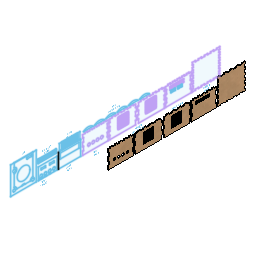
cardboard_box_v3 (Autodesk Fusion 360 design; units mm, degrees)
Autodesk Fusion 360 part; units mm, degrees
(part 1 of 3)
sketch "bottom sketch" plane through (0, 0, 0) normal (0, 0, 1) x (1, 0, 0)
  line L0 (0, 0) -> (150, 0)
  line L1 (150, 0) -> (150, 161)
  line L2 (150, 161) -> (0, 161)
  line L3 (0, 161) -> (0, 0)
  dimension "d9" = 150
  dimension "d10" = 161
  constraint horizontal L0
  constraint vertical L1
  constraint horizontal L2
  constraint vertical L3
  constraint coincident L0.start L3.end
  measures "d9" distance of L0.start L0.end
  measures "d10" distance of L0.start L2.end
extrude "Extrude1" add sketch "bottom sketch" along normal blind 5 makes body 1
sketch "bottom panel front fingers sketch" plane through (0, 0, 0) normal (0, -1, 0) x (1, 0, 0)
  line L0 (0, 0) -> (150, 0)
  line L1 (150, 0) -> (150, 5)
  line L2 (150, 5) -> (0, 5)
  line L3 (0, 5) -> (0, 0)
  line L4 (13.6364, 0) -> (27.2727, 0)
  line L5 (27.2727, 0) -> (27.2727, 5)
  line L6 (27.2727, 5) -> (13.6364, 5)
  line L7 (13.6364, 5) -> (13.6364, 0)
  dimension "d19" = 13.6364
  dimension "d20" = 13.6364
  constraint horizontal L4
  constraint vertical L5
  constraint horizontal L6
  constraint vertical L7
  constraint coincident L2 L5.end
  constraint coincident L0 L4.start
  measures "d19" distance of L5.end L6.end
  measures "d20" distance of L3 L7
extrude "Extrude2" cut sketch "bottom panel front fingers sketch" against normal blind 5 contours L0 L2 L4 L5 L6 L7 bodies 1
pattern_linear "R-Pattern1" count 5 spacing 27.2727 along (1, 0, 0) of "Extrude2"
sketch "front panel sketch" plane through (0, 0, 0) normal (0, 1, 0) x (1, 0, 0)
  line L0 (0, 0) -> (150, 0)
  line L1 (150, 0) -> (150, -110)
  line L2 (150, -110) -> (0, -110)
  line L3 (0, -110) -> (0, 0)
  dimension "d27" = 110
  constraint perpendicular L0 L1
  constraint parallel L0 L2
  constraint parallel L1 L3
  constraint horizontal L0
  constraint coincident L0.start L3.end
  measures "d27" distance of L0.start L2.end
extrude "Extrude3" add sketch "front panel sketch" along normal blind 5 separate body makes body 2
combine "Combine1" operation cut target body 2 tool bodies 1 keep tools
sketch "front panel left finger sketch" plane through (0, 0, 0) normal (-1, 0, 0) x (0, -1, 0)
  line L0 (-5, 5) -> (0, 5)
  line L1 (0, 5) -> (0, 110)
  line L2 (0, 110) -> (-5, 110)
  line L3 (-5, 110) -> (-5, 5)
  line L4 (0, 22) -> (-5, 22)
  line L5 (-5, 22) -> (-5, 44)
  line L6 (-5, 44) -> (0, 44)
  line L7 (0, 44) -> (0, 22)
  dimension "d30" = 22
  dimension "d31" = 22
  constraint horizontal L4
  constraint vertical L5
  constraint horizontal L6
  constraint vertical L7
  constraint coincident L3 L5.end
  constraint coincident L1 L4.start
  measures "d30" distance of L4.start L6.end
  measures "d31" distance of L4.start origin
extrude "Extrude4" cut sketch "front panel left finger sketch" against normal blind 5 contours L1 L3 L4 L5 L6 L7 bodies 2
pattern_linear "R-Pattern2" count 1 spacing 0 along (1, 0, 0) count 2 spacing 44 along (0, 0, 1) of "Extrude4"
extrude "Extrude5" add 1 faces at (78.9394, 5, 67.6667) along direction (0, -1, 0) blind 5 from surface at -156 separate body on bodies 2 makes body 3
combine "Combine2" operation cut target body 1 tool bodies 3 keep tools
sketch "left panel sketch" plane through (0, 0, 0) normal (1, 0, 0) x (0, 1, 0)
  line L0 (161, 0) -> (0, 0)
  line L1 (0, 0) -> (0, 110)
  line L2 (0, 110) -> (161, 110)
  line L3 (161, 110) -> (161, 0)
  line L4 (107.3333, 82.5) -> (101.3333, 82.5)
  line L5 (101.3333, 82.5) -> (101.3333, 76.5)
  line L6 (101.3333, 76.5) -> (107.3333, 76.5)
  line L7 (107.3333, 76.5) -> (107.3333, 82.5)
  dimension "d54" = 161
  dimension "d55" = 6
  dimension "d56" = 6
  dimension "d57" = 53.6667
  dimension "d66" = 27.5
  constraint perpendicular L0 L1
  constraint parallel L0 L2
  constraint parallel L1 L3
  constraint coincident L0.end L1.start
  constraint horizontal L0
  constraint horizontal L4
  constraint vertical L5
  constraint horizontal L6
  constraint vertical L7
  measures "d54" distance of L1.end L2.end
  measures "d55" distance of L4.start L4.end
  measures "d56" distance of L4.start L6.end
  measures "d57" distance of L3 L7
  measures "d66" distance of L2 L4
extrude "Extrude6" add sketch "left panel sketch" along normal blind 5 separate body contours L0 L1 L2 L3 | L4 L5 L6 L7 makes body 4
sketch "bottom panel left finger sketch" plane through (0, 0, 0) normal (-1, 0, 0) x (0, -1, 0)
  line L0 (-161, 0) -> (0, 0)
  line L1 (0, 0) -> (0, 5)
  line L2 (0, 5) -> (-161, 5)
  line L3 (-161, 5) -> (-161, 0)
  line L4 (-35.7778, 0) -> (-17.8889, 0)
  line L5 (-17.8889, 0) -> (-17.8889, 5)
  line L6 (-17.8889, 5) -> (-35.7778, 5)
  line L7 (-35.7778, 5) -> (-35.7778, 0)
  dimension "d43" = 17.8889
  dimension "d44" = 17.8889
  constraint horizontal L4
  constraint vertical L5
  constraint horizontal L6
  constraint vertical L7
  constraint coincident L2 L5.end
  constraint coincident L0 L4.start
  measures "d43" distance of L4.start L4.end
  measures "d44" distance of L1 L5
extrude "Extrude7" cut sketch "bottom panel left finger sketch" against normal blind 5 contours L0 L2 L4 L5 L6 L7 bodies 1
pattern_linear "R-Pattern3" count 4 spacing 35.7778 along (0, 1, 0) of "Extrude7"
combine "Combine3" operation cut target body 4 tool bodies 2 1 3 keep tools
extrude "Extrude9" cut sketch "left panel sketch" along normal blind 150 contours L4 L5 L6 L7 bodies 4
pattern_linear "R-Pattern4" count 8 spacing 7.6667 along (0, -1, 0) count 8 spacing 7.8571 along (0, 0, -1) of "Extrude9"
extrude "Extrude10" add 1 faces at (5, 84.3333, 100.8333) along direction (-1, 0, 0) blind 5 from surface at -145 separate body on bodies 4 makes body 5
combine "Combine7" operation cut target body 2 tool bodies 5 keep tools
combine "Combine8" operation cut target body 1 tool bodies 5 keep tools
combine "Combine9" operation cut target body 3 tool bodies 5 keep tools
sketch "Sketch7" plane through (0, 0, 0) normal (0, -1, 0) x (1, 0, 0)
  line L0 (145, 88) -> (150, 88)
  line L1 (150, 88) -> (150, 110)
  line L2 (150, 110) -> (0, 110)
  line L3 (0, 110) -> (0, 88)
  line L4 (0, 88) -> (5, 88)
  line L5 (5, 88) -> (5, 66)
  line L6 (5, 66) -> (0, 66)
  line L7 (0, 66) -> (0, 44)
  line L8 (0, 44) -> (5, 44)
  line L9 (5, 44) -> (5, 22)
  line L10 (5, 22) -> (0, 22)
  line L11 (0, 22) -> (0, 5)
  line L12 (0, 5) -> (13.6364, 5)
  line L13 (13.6364, 5) -> (13.6364, 0)
  line L14 (13.6364, 0) -> (27.2727, 0)
  line L15 (27.2727, 0) -> (27.2727, 5)
  line L16 (27.2727, 5) -> (40.9091, 5)
  line L17 (40.9091, 5) -> (40.9091, 0)
  line L18 (40.9091, 0) -> (54.5455, 0)
  line L19 (54.5455, 0) -> (54.5455, 5)
  line L20 (54.5455, 5) -> (68.1818, 5)
  line L21 (68.1818, 5) -> (68.1818, 0)
  line L22 (68.1818, 0) -> (81.8182, 0)
  line L23 (81.8182, 0) -> (81.8182, 5)
  line L24 (81.8182, 5) -> (95.4545, 5)
  line L25 (95.4545, 5) -> (95.4545, 0)
  line L26 (95.4545, 0) -> (109.0909, 0)
  line L27 (109.0909, 0) -> (109.0909, 5)
  line L28 (109.0909, 5) -> (122.7273, 5)
  line L29 (122.7273, 5) -> (122.7273, 0)
  line L30 (122.7273, 0) -> (136.3636, 0)
  line L31 (136.3636, 0) -> (136.3636, 5)
  line L32 (136.3636, 5) -> (150, 5)
  line L33 (150, 5) -> (150, 22)
  line L34 (150, 22) -> (145, 22)
  line L35 (145, 22) -> (145, 44)
  line L36 (145, 44) -> (150, 44)
  line L37 (150, 44) -> (150, 66)
  line L38 (150, 66) -> (145, 66)
  line L39 (145, 66) -> (145, 88)
  circle A0 centre (37.5, 73.3333) radius 7.5
  dimension "d70" = 15
  dimension "d71" = 37.5
  dimension "d72" = 36.6667
  measures "d70" diameter of A0
  measures "d71" distance of L3 A0.centre
  measures "d72" distance of L2 A0.centre
extrude "Extrude11" cut sketch "Sketch7" against normal blind 5 contours A0 bodies 2
pattern_linear "R-Pattern5" count 4 spacing 25 along (1, 0, 0) of "Extrude11"
sketch "Sketch8" plane through (0, 161, 0) normal (0, 1, 0) x (-1, 0, 0)
  line L0 (-145, 22) -> (-150, 22)
  line L1 (-150, 22) -> (-150, 5)
  line L2 (-150, 5) -> (-136.3636, 5)
  line L3 (-136.3636, 5) -> (-136.3636, 0)
  line L4 (-136.3636, 0) -> (-122.7273, 0)
  line L5 (-122.7273, 0) -> (-122.7273, 5)
  line L6 (-122.7273, 5) -> (-109.0909, 5)
  line L7 (-109.0909, 5) -> (-109.0909, 0)
  line L8 (-109.0909, 0) -> (-95.4545, 0)
  line L9 (-95.4545, 0) -> (-95.4545, 5)
  line L10 (-95.4545, 5) -> (-81.8182, 5)
  line L11 (-81.8182, 5) -> (-81.8182, 0)
  line L12 (-81.8182, 0) -> (-68.1818, 0)
  line L13 (-68.1818, 0) -> (-68.1818, 5)
  line L14 (-68.1818, 5) -> (-54.5455, 5)
  line L15 (-54.5455, 5) -> (-54.5455, 0)
  line L16 (-54.5455, 0) -> (-40.9091, 0)
  line L17 (-40.9091, 0) -> (-40.9091, 5)
  line L18 (-40.9091, 5) -> (-27.2727, 5)
  line L19 (-27.2727, 5) -> (-27.2727, 0)
  line L20 (-27.2727, 0) -> (-13.6364, 0)
  line L21 (-13.6364, 0) -> (-13.6364, 5)
  line L22 (-13.6364, 5) -> (0, 5)
  line L23 (0, 5) -> (0, 22)
  line L24 (0, 22) -> (-5, 22)
  line L25 (-5, 22) -> (-5, 44)
  line L26 (-5, 44) -> (0, 44)
  line L27 (0, 44) -> (0, 66)
  line L28 (0, 66) -> (-5, 66)
  line L29 (-5, 66) -> (-5, 88)
  line L30 (-5, 88) -> (0, 88)
  line L31 (0, 88) -> (0, 110)
  line L32 (0, 110) -> (-150, 110)
  line L33 (-150, 110) -> (-150, 88)
  line L34 (-150, 88) -> (-145, 88)
  line L35 (-145, 88) -> (-145, 66)
  line L36 (-145, 66) -> (-150, 66)
  line L37 (-150, 66) -> (-150, 44)
  line L38 (-150, 44) -> (-145, 44)
  line L39 (-145, 44) -> (-145, 22)
  line L40 (-31, 33.3333) -> (-25, 33.3333)
  line L41 (-25, 33.3333) -> (-25, 18.3333)
  line L42 (-25, 18.3333) -> (-31, 18.3333)
  line L43 (-31, 18.3333) -> (-31, 33.3333)
  dimension "d79" = 6
  dimension "d80" = 15
  dimension "d81" = 18.3333
  dimension "d82" = 25
  constraint horizontal L40
  constraint vertical L41
  constraint horizontal L42
  constraint vertical L43
  measures "d79" distance of L40.start L40.end
  measures "d80" distance of L40.end L41.end
  measures "d81" distance of L20 L42
  measures "d82" distance of L23.end L41
extrude "Extrude12" cut sketch "Sketch8" against normal blind 5 contours L40 L41 L42 L43 bodies 3
pattern_linear "R-Pattern6" count 10 spacing 8.3333 along (1, 0, 0) of "Extrude12"
copy_body "Body->Comp1" bodies 5 removing the originals makes body 6 in component "right panel"
copy_body "Body->Comp2" bodies 2 removing the originals makes body 7 in component "front panel"
copy_body "Body->Comp3" bodies 1 removing the originals makes body 8 in component "bottom panel"
copy_body "Body->Comp4" bodies 3 removing the originals makes body 9 in component "back panel"
copy_body "Body->Comp5" bodies 4 removing the originals makes body 10 in component "left panel"
move_face "MoveFace1" by (0, 0, 10) 1 faces at (150, 84.3333, 100.8333) on bodies 6 in component "right panel"
move_body "Move1" bodies 6 to x (1, 0, 0) y (0, 1, 0) z (0, 0, 1) at (0, 0, 5) in component "right panel"
move_face "MoveFace1'" by (0, 0, 5) 1 faces at (75, 161, 69.7778) on bodies 9 in component "back panel"
move_body "Move1'" bodies 10 to x (1, 0, 0) y (0, 1, 0) z (0, 0, 1) at (0, 0, 5) in component "left panel"
move_body "Move1''" bodies 7 to x (1, 0, 0) y (0, 1, 0) z (0, 0, 1) at (0, 0, 5) in component "front panel"
move_body "Move1'''" bodies 9 to x (1, 0, 0) y (0, 1, 0) z (0, 0, 1) at (0, 0, 5) in component "back panel"
move_body "Move2" bodies 9 to x (0, 0, 1) y (0, 1, 0) z (-1, 0, 0) at (19.7108, 0, -5.5056) in component "back panel"
move_body "Move3" bodies 9 to x (1, 0, 0) y (0, 1, 0) z (0, 0, 1) at (-20.3452, 0, 10.1726) in component "back panel"
move_body "Move2'" bodies 6 to x (1, 0, 0) y (0, -1, 0) z (0, 0, -1) at (0, -7.1131, -149.8096) in component "right panel"
move_body "Move2''" bodies 7 to x (0, 0, 1) y (0, 1, 0) z (-1, 0, 0) at (-0.3493, 0, 172.3854) in component "front panel"
move_body "Move1''''" bodies 8 to x (1, 0, 0) y (0, 1, 0) z (0, 0, 1) at (-116.6753, 330.7142, 0) in component "bottom panel"
sketch "Sketch10" plane through (150, 0, 0) normal (1, 0, 0) x (0, 1, 0)
  line L0 (53.6667, -182.5) -> (47.6667, -182.5)
  line L1 (47.6667, -182.5) -> (47.6667, -176.5)
  line L2 (47.6667, -176.5) -> (53.6667, -176.5)
  line L3 (53.6667, -176.5) -> (53.6667, -182.5)
  line L4 (61.3333, -182.5) -> (55.3333, -182.5)
  line L5 (55.3333, -182.5) -> (55.3333, -176.5)
  line L6 (55.3333, -176.5) -> (61.3333, -176.5)
  line L7 (61.3333, -176.5) -> (61.3333, -182.5)
  line L8 (69, -182.5) -> (63, -182.5)
  line L9 (63, -182.5) -> (63, -176.5)
  line L10 (63, -176.5) -> (69, -176.5)
  line L11 (69, -176.5) -> (69, -182.5)
  line L12 (76.6667, -182.5) -> (70.6667, -182.5)
  line L13 (70.6667, -182.5) -> (70.6667, -176.5)
  line L14 (70.6667, -176.5) -> (76.6667, -176.5)
  line L15 (76.6667, -176.5) -> (76.6667, -182.5)
  line L16 (84.3333, -182.5) -> (78.3333, -182.5)
  line L17 (78.3333, -182.5) -> (78.3333, -176.5)
  line L18 (78.3333, -176.5) -> (84.3333, -176.5)
  line L19 (84.3333, -176.5) -> (84.3333, -182.5)
  line L20 (92, -182.5) -> (86, -182.5)
  line L21 (86, -182.5) -> (86, -176.5)
  line L22 (86, -176.5) -> (92, -176.5)
  line L23 (92, -176.5) -> (92, -182.5)
  line L24 (99.6667, -182.5) -> (93.6667, -182.5)
  line L25 (93.6667, -182.5) -> (93.6667, -176.5)
  line L26 (93.6667, -176.5) -> (99.6667, -176.5)
  line L27 (99.6667, -176.5) -> (99.6667, -182.5)
  line L28 (107.3333, -182.5) -> (101.3333, -182.5)
  line L29 (101.3333, -182.5) -> (101.3333, -176.5)
  line L30 (101.3333, -176.5) -> (107.3333, -176.5)
  line L31 (107.3333, -176.5) -> (107.3333, -182.5)
  line L32 (53.6667, -190.3571) -> (47.6667, -190.3571)
  line L33 (47.6667, -190.3571) -> (47.6667, -184.3571)
  line L34 (47.6667, -184.3571) -> (53.6667, -184.3571)
  line L35 (53.6667, -184.3571) -> (53.6667, -190.3571)
  line L36 (61.3333, -190.3571) -> (55.3333, -190.3571)
  line L37 (55.3333, -190.3571) -> (55.3333, -184.3571)
  line L38 (55.3333, -184.3571) -> (61.3333, -184.3571)
  line L39 (61.3333, -184.3571) -> (61.3333, -190.3571)
  line L40 (69, -190.3571) -> (63, -190.3571)
  line L41 (63, -190.3571) -> (63, -184.3571)
  line L42 (63, -184.3571) -> (69, -184.3571)
  line L43 (69, -184.3571) -> (69, -190.3571)
  line L44 (76.6667, -190.3571) -> (70.6667, -190.3571)
  line L45 (70.6667, -190.3571) -> (70.6667, -184.3571)
  line L46 (70.6667, -184.3571) -> (76.6667, -184.3571)
  line L47 (76.6667, -184.3571) -> (76.6667, -190.3571)
  line L48 (84.3333, -190.3571) -> (78.3333, -190.3571)
  line L49 (78.3333, -190.3571) -> (78.3333, -184.3571)
  line L50 (78.3333, -184.3571) -> (84.3333, -184.3571)
  line L51 (84.3333, -184.3571) -> (84.3333, -190.3571)
  line L52 (92, -190.3571) -> (86, -190.3571)
  line L53 (86, -190.3571) -> (86, -184.3571)
  line L54 (86, -184.3571) -> (92, -184.3571)
  line L55 (92, -184.3571) -> (92, -190.3571)
  line L56 (99.6667, -190.3571) -> (93.6667, -190.3571)
  line L57 (93.6667, -190.3571) -> (93.6667, -184.3571)
  line L58 (93.6667, -184.3571) -> (99.6667, -184.3571)
  line L59 (99.6667, -184.3571) -> (99.6667, -190.3571)
  line L60 (107.3333, -190.3571) -> (101.3333, -190.3571)
  line L61 (101.3333, -190.3571) -> (101.3333, -184.3571)
  line L62 (101.3333, -184.3571) -> (107.3333, -184.3571)
  line L63 (107.3333, -184.3571) -> (107.3333, -190.3571)
  line L64 (53.6667, -198.2143) -> (47.6667, -198.2143)
  line L65 (47.6667, -198.2143) -> (47.6667, -192.2143)
  line L66 (47.6667, -192.2143) -> (53.6667, -192.2143)
  line L67 (53.6667, -192.2143) -> (53.6667, -198.2143)
  line L68 (61.3333, -198.2143) -> (55.3333, -198.2143)
  line L69 (55.3333, -198.2143) -> (55.3333, -192.2143)
  line L70 (55.3333, -192.2143) -> (61.3333, -192.2143)
  line L71 (61.3333, -192.2143) -> (61.3333, -198.2143)
  line L72 (69, -198.2143) -> (63, -198.2143)
  line L73 (63, -198.2143) -> (63, -192.2143)
  line L74 (63, -192.2143) -> (69, -192.2143)
  line L75 (69, -192.2143) -> (69, -198.2143)
  line L76 (76.6667, -198.2143) -> (70.6667, -198.2143)
  line L77 (70.6667, -198.2143) -> (70.6667, -192.2143)
  line L78 (70.6667, -192.2143) -> (76.6667, -192.2143)
  line L79 (76.6667, -192.2143) -> (76.6667, -198.2143)
  line L80 (84.3333, -198.2143) -> (78.3333, -198.2143)
  line L81 (78.3333, -198.2143) -> (78.3333, -192.2143)
  line L82 (78.3333, -192.2143) -> (84.3333, -192.2143)
  line L83 (84.3333, -192.2143) -> (84.3333, -198.2143)
  line L84 (92, -198.2143) -> (86, -198.2143)
  line L85 (86, -198.2143) -> (86, -192.2143)
  line L86 (86, -192.2143) -> (92, -192.2143)
  line L87 (92, -192.2143) -> (92, -198.2143)
  line L88 (99.6667, -198.2143) -> (93.6667, -198.2143)
  line L89 (93.6667, -198.2143) -> (93.6667, -192.2143)
  line L90 (93.6667, -192.2143) -> (99.6667, -192.2143)
  line L91 (99.6667, -192.2143) -> (99.6667, -198.2143)
  line L92 (107.3333, -198.2143) -> (101.3333, -198.2143)
  line L93 (101.3333, -198.2143) -> (101.3333, -192.2143)
  line L94 (101.3333, -192.2143) -> (107.3333, -192.2143)
  line L95 (107.3333, -192.2143) -> (107.3333, -198.2143)
  line L96 (53.6667, -206.0714) -> (47.6667, -206.0714)
  line L97 (47.6667, -206.0714) -> (47.6667, -200.0714)
  line L98 (47.6667, -200.0714) -> (53.6667, -200.0714)
  line L99 (53.6667, -200.0714) -> (53.6667, -206.0714)
  line L100 (61.3333, -206.0714) -> (55.3333, -206.0714)
  line L101 (55.3333, -206.0714) -> (55.3333, -200.0714)
  line L102 (55.3333, -200.0714) -> (61.3333, -200.0714)
  line L103 (61.3333, -200.0714) -> (61.3333, -206.0714)
  line L104 (69, -206.0714) -> (63, -206.0714)
  line L105 (63, -206.0714) -> (63, -200.0714)
  line L106 (63, -200.0714) -> (69, -200.0714)
  line L107 (69, -200.0714) -> (69, -206.0714)
  line L108 (76.6667, -206.0714) -> (70.6667, -206.0714)
  line L109 (70.6667, -206.0714) -> (70.6667, -200.0714)
  line L110 (70.6667, -200.0714) -> (76.6667, -200.0714)
  line L111 (76.6667, -200.0714) -> (76.6667, -206.0714)
  line L112 (84.3333, -206.0714) -> (78.3333, -206.0714)
  line L113 (78.3333, -206.0714) -> (78.3333, -200.0714)
  line L114 (78.3333, -200.0714) -> (84.3333, -200.0714)
  line L115 (84.3333, -200.0714) -> (84.3333, -206.0714)
  line L116 (92, -206.0714) -> (86, -206.0714)
  line L117 (86, -206.0714) -> (86, -200.0714)
  line L118 (86, -200.0714) -> (92, -200.0714)
  line L119 (92, -200.0714) -> (92, -206.0714)
  line L120 (99.6667, -206.0714) -> (93.6667, -206.0714)
  line L121 (93.6667, -206.0714) -> (93.6667, -200.0714)
  line L122 (93.6667, -200.0714) -> (99.6667, -200.0714)
  line L123 (99.6667, -200.0714) -> (99.6667, -206.0714)
  line L124 (107.3333, -206.0714) -> (101.3333, -206.0714)
  line L125 (101.3333, -206.0714) -> (101.3333, -200.0714)
  line L126 (101.3333, -200.0714) -> (107.3333, -200.0714)
  line L127 (107.3333, -200.0714) -> (107.3333, -206.0714)
  line L128 (53.6667, -213.9286) -> (47.6667, -213.9286)
  line L129 (47.6667, -213.9286) -> (47.6667, -207.9286)
  line L130 (47.6667, -207.9286) -> (53.6667, -207.9286)
  line L131 (53.6667, -207.9286) -> (53.6667, -213.9286)
  line L132 (61.3333, -213.9286) -> (55.3333, -213.9286)
  line L133 (55.3333, -213.9286) -> (55.3333, -207.9286)
  line L134 (55.3333, -207.9286) -> (61.3333, -207.9286)
  line L135 (61.3333, -207.9286) -> (61.3333, -213.9286)
  line L136 (69, -213.9286) -> (63, -213.9286)
  line L137 (63, -213.9286) -> (63, -207.9286)
  line L138 (63, -207.9286) -> (69, -207.9286)
  line L139 (69, -207.9286) -> (69, -213.9286)
  line L140 (76.6667, -213.9286) -> (70.6667, -213.9286)
  line L141 (70.6667, -213.9286) -> (70.6667, -207.9286)
  line L142 (70.6667, -207.9286) -> (76.6667, -207.9286)
  line L143 (76.6667, -207.9286) -> (76.6667, -213.9286)
  line L144 (84.3333, -213.9286) -> (78.3333, -213.9286)
  line L145 (78.3333, -213.9286) -> (78.3333, -207.9286)
  line L146 (78.3333, -207.9286) -> (84.3333, -207.9286)
  line L147 (84.3333, -207.9286) -> (84.3333, -213.9286)
  line L148 (92, -213.9286) -> (86, -213.9286)
  line L149 (86, -213.9286) -> (86, -207.9286)
  line L150 (86, -207.9286) -> (92, -207.9286)
  line L151 (92, -207.9286) -> (92, -213.9286)
  line L152 (99.6667, -213.9286) -> (93.6667, -213.9286)
  line L153 (93.6667, -213.9286) -> (93.6667, -207.9286)
  line L154 (93.6667, -207.9286) -> (99.6667, -207.9286)
  line L155 (99.6667, -207.9286) -> (99.6667, -213.9286)
  line L156 (107.3333, -213.9286) -> (101.3333, -213.9286)
  line L157 (101.3333, -213.9286) -> (101.3333, -207.9286)
  line L158 (101.3333, -207.9286) -> (107.3333, -207.9286)
  line L159 (107.3333, -207.9286) -> (107.3333, -213.9286)
  line L160 (53.6667, -221.7857) -> (47.6667, -221.7857)
  line L161 (47.6667, -221.7857) -> (47.6667, -215.7857)
  line L162 (47.6667, -215.7857) -> (53.6667, -215.7857)
  line L163 (53.6667, -215.7857) -> (53.6667, -221.7857)
  line L164 (61.3333, -221.7857) -> (55.3333, -221.7857)
  line L165 (55.3333, -221.7857) -> (55.3333, -215.7857)
  line L166 (55.3333, -215.7857) -> (61.3333, -215.7857)
  line L167 (61.3333, -215.7857) -> (61.3333, -221.7857)
  line L168 (69, -221.7857) -> (63, -221.7857)
  line L169 (63, -221.7857) -> (63, -215.7857)
  line L170 (63, -215.7857) -> (69, -215.7857)
  line L171 (69, -215.7857) -> (69, -221.7857)
  line L172 (76.6667, -221.7857) -> (70.6667, -221.7857)
  line L173 (70.6667, -221.7857) -> (70.6667, -215.7857)
  line L174 (70.6667, -215.7857) -> (76.6667, -215.7857)
  line L175 (76.6667, -215.7857) -> (76.6667, -221.7857)
  line L176 (84.3333, -221.7857) -> (78.3333, -221.7857)
  line L177 (78.3333, -221.7857) -> (78.3333, -215.7857)
  line L178 (78.3333, -215.7857) -> (84.3333, -215.7857)
  line L179 (84.3333, -215.7857) -> (84.3333, -221.7857)
  line L180 (92, -221.7857) -> (86, -221.7857)
  line L181 (86, -221.7857) -> (86, -215.7857)
  line L182 (86, -215.7857) -> (92, -215.7857)
  line L183 (92, -215.7857) -> (92, -221.7857)
  line L184 (99.6667, -221.7857) -> (93.6667, -221.7857)
  line L185 (93.6667, -221.7857) -> (93.6667, -215.7857)
  line L186 (93.6667, -215.7857) -> (99.6667, -215.7857)
  line L187 (99.6667, -215.7857) -> (99.6667, -221.7857)
  line L188 (107.3333, -221.7857) -> (101.3333, -221.7857)
  line L189 (101.3333, -221.7857) -> (101.3333, -215.7857)
  line L190 (101.3333, -215.7857) -> (107.3333, -215.7857)
  line L191 (107.3333, -215.7857) -> (107.3333, -221.7857)
  line L192 (53.6667, -229.6429) -> (47.6667, -229.6429)
  line L193 (47.6667, -229.6429) -> (47.6667, -223.6429)
  line L194 (47.6667, -223.6429) -> (53.6667, -223.6429)
  line L195 (53.6667, -223.6429) -> (53.6667, -229.6429)
  line L196 (61.3333, -229.6429) -> (55.3333, -229.6429)
  line L197 (55.3333, -229.6429) -> (55.3333, -223.6429)
  line L198 (55.3333, -223.6429) -> (61.3333, -223.6429)
  line L199 (61.3333, -223.6429) -> (61.3333, -229.6429)
  line L200 (69, -229.6429) -> (63, -229.6429)
  line L201 (63, -229.6429) -> (63, -223.6429)
  line L202 (63, -223.6429) -> (69, -223.6429)
  line L203 (69, -223.6429) -> (69, -229.6429)
  line L204 (76.6667, -229.6429) -> (70.6667, -229.6429)
  line L205 (70.6667, -229.6429) -> (70.6667, -223.6429)
  line L206 (70.6667, -223.6429) -> (76.6667, -223.6429)
  line L207 (76.6667, -223.6429) -> (76.6667, -229.6429)
  line L208 (84.3333, -229.6429) -> (78.3333, -229.6429)
  line L209 (78.3333, -229.6429) -> (78.3333, -223.6429)
  line L210 (78.3333, -223.6429) -> (84.3333, -223.6429)
  line L211 (84.3333, -223.6429) -> (84.3333, -229.6429)
  line L212 (92, -229.6429) -> (86, -229.6429)
  line L213 (86, -229.6429) -> (86, -223.6429)
  line L214 (86, -223.6429) -> (92, -223.6429)
  line L215 (92, -223.6429) -> (92, -229.6429)
  line L216 (99.6667, -229.6429) -> (93.6667, -229.6429)
  line L217 (93.6667, -229.6429) -> (93.6667, -223.6429)
  line L218 (93.6667, -223.6429) -> (99.6667, -223.6429)
  line L219 (99.6667, -223.6429) -> (99.6667, -229.6429)
  line L220 (107.3333, -229.6429) -> (101.3333, -229.6429)
  line L221 (101.3333, -229.6429) -> (101.3333, -223.6429)
  line L222 (101.3333, -223.6429) -> (107.3333, -223.6429)
  line L223 (107.3333, -223.6429) -> (107.3333, -229.6429)
  line L224 (53.6667, -237.5) -> (47.6667, -237.5)
  line L225 (47.6667, -237.5) -> (47.6667, -231.5)
  line L226 (47.6667, -231.5) -> (53.6667, -231.5)
  line L227 (53.6667, -231.5) -> (53.6667, -237.5)
  line L228 (61.3333, -237.5) -> (55.3333, -237.5)
  line L229 (55.3333, -237.5) -> (55.3333, -231.5)
  line L230 (55.3333, -231.5) -> (61.3333, -231.5)
  line L231 (61.3333, -231.5) -> (61.3333, -237.5)
  line L232 (69, -237.5) -> (63, -237.5)
  line L233 (63, -237.5) -> (63, -231.5)
  line L234 (63, -231.5) -> (69, -231.5)
  line L235 (69, -231.5) -> (69, -237.5)
  line L236 (76.6667, -237.5) -> (70.6667, -237.5)
  line L237 (70.6667, -237.5) -> (70.6667, -231.5)
  line L238 (70.6667, -231.5) -> (76.6667, -231.5)
  line L239 (76.6667, -231.5) -> (76.6667, -237.5)
  line L240 (84.3333, -237.5) -> (78.3333, -237.5)
  line L241 (78.3333, -237.5) -> (78.3333, -231.5)
  line L242 (78.3333, -231.5) -> (84.3333, -231.5)
  line L243 (84.3333, -231.5) -> (84.3333, -237.5)
  line L244 (92, -237.5) -> (86, -237.5)
  line L245 (86, -237.5) -> (86, -231.5)
  line L246 (86, -231.5) -> (92, -231.5)
  line L247 (92, -231.5) -> (92, -237.5)
  line L248 (99.6667, -237.5) -> (93.6667, -237.5)
  line L249 (93.6667, -237.5) -> (93.6667, -231.5)
  line L250 (93.6667, -231.5) -> (99.6667, -231.5)
  line L251 (99.6667, -231.5) -> (99.6667, -237.5)
  line L252 (101.3333, -231.5) -> (107.3333, -231.5)
  line L253 (107.3333, -231.5) -> (107.3333, -237.5)
  line L254 (107.3333, -237.5) -> (101.3333, -237.5)
  line L255 (101.3333, -237.5) -> (101.3333, -231.5)
  line L256 (156, -177) -> (156, -160)
  line L257 (156, -160) -> (143.1111, -160)
  line L258 (143.1111, -160) -> (143.1111, -155)
  line L259 (143.1111, -155) -> (125.2222, -155)
  line L260 (125.2222, -155) -> (125.2222, -160)
  line L261 (125.2222, -160) -> (107.3333, -160)
  line L262 (107.3333, -160) -> (107.3333, -155)
  line L263 (107.3333, -155) -> (89.4444, -155)
  line L264 (89.4444, -155) -> (89.4444, -160)
  line L265 (89.4444, -160) -> (71.5556, -160)
  line L266 (71.5556, -160) -> (71.5556, -155)
  line L267 (71.5556, -155) -> (53.6667, -155)
  line L268 (53.6667, -155) -> (53.6667, -160)
  line L269 (53.6667, -160) -> (35.7778, -160)
  line L270 (35.7778, -160) -> (35.7778, -155)
  line L271 (35.7778, -155) -> (17.8889, -155)
  line L272 (17.8889, -155) -> (17.8889, -160)
  line L273 (17.8889, -160) -> (5, -160)
  line L274 (5, -160) -> (5, -177)
  line L275 (5, -177) -> (0, -177)
  line L276 (0, -177) -> (0, -199)
  line L277 (0, -199) -> (5, -199)
  line L278 (5, -199) -> (5, -221)
  line L279 (5, -221) -> (0, -221)
  line L280 (0, -221) -> (0, -243)
  line L281 (0, -243) -> (5, -243)
  line L282 (5, -243) -> (5, -265)
  line L283 (5, -265) -> (156, -265)
  line L284 (156, -265) -> (156, -243)
  line L285 (156, -243) -> (161, -243)
  line L286 (161, -243) -> (161, -221)
  line L287 (161, -221) -> (156, -221)
  line L288 (156, -221) -> (156, -199)
  line L289 (156, -199) -> (161, -199)
  line L290 (161, -199) -> (161, -177)
  line L291 (161, -177) -> (156, -177)
move_body "Move4" bodies 9 to x (1, 0, 0) y (0, 1, 0) z (0, 0, 1) at (1.319, 0, -1.319) in component "back panel"
move_body "Move2'''" bodies 8 to x (1, 0, 0) y (0, 1, 0) z (0, 0, 1) at (2.6379, -10.2219, 0) in component "bottom panel"
move_body "Move3'" bodies 6 to x (1, 0, 0) y (0, 1, 0) z (0, 0, 1) at (0, 0, 0.3297) in component "right panel"
move_body "Move3''" bodies 7 to x (1, 0, 0) y (0, 1, 0) z (0, 0, 1) at (0.6595, 0, 0.3297) in component "front panel"
sketch "Sketch11" plane through (150, 0, 0) normal (1, 0, 0) x (0, 1, 0)
  circle A0 centre (-285.2151, -228.0231) radius 7.5
  circle A1 centre (-260.2151, -228.0231) radius 7.5
  circle A2 centre (-235.2151, -228.0231) radius 7.5
  circle A3 centre (-210.2151, -228.0231) radius 7.5
  line L0 (-317.7151, -242.6898) -> (-322.7151, -242.6898)
  line L1 (-322.7151, -242.6898) -> (-322.7151, -264.6898)
  line L2 (-322.7151, -264.6898) -> (-172.7151, -264.6898)
  line L3 (-172.7151, -264.6898) -> (-172.7151, -242.6898)
  line L4 (-172.7151, -242.6898) -> (-177.7151, -242.6898)
  line L5 (-177.7151, -242.6898) -> (-177.7151, -220.6898)
  line L6 (-177.7151, -220.6898) -> (-172.7151, -220.6898)
  line L7 (-172.7151, -220.6898) -> (-172.7151, -198.6898)
  line L8 (-172.7151, -198.6898) -> (-177.7151, -198.6898)
  line L9 (-177.7151, -198.6898) -> (-177.7151, -176.6898)
  line L10 (-177.7151, -176.6898) -> (-172.7151, -176.6898)
  line L11 (-172.7151, -176.6898) -> (-172.7151, -159.6898)
  line L12 (-172.7151, -159.6898) -> (-186.3515, -159.6898)
  line L13 (-186.3515, -159.6898) -> (-186.3515, -154.6898)
  line L14 (-186.3515, -154.6898) -> (-199.9879, -154.6898)
  line L15 (-199.9879, -154.6898) -> (-199.9879, -159.6898)
  line L16 (-199.9879, -159.6898) -> (-213.6242, -159.6898)
  line L17 (-213.6242, -159.6898) -> (-213.6242, -154.6898)
  line L18 (-213.6242, -154.6898) -> (-227.2606, -154.6898)
  line L19 (-227.2606, -154.6898) -> (-227.2606, -159.6898)
  line L20 (-227.2606, -159.6898) -> (-240.897, -159.6898)
  line L21 (-240.897, -159.6898) -> (-240.897, -154.6898)
  line L22 (-240.897, -154.6898) -> (-254.5333, -154.6898)
  line L23 (-254.5333, -154.6898) -> (-254.5333, -159.6898)
  line L24 (-254.5333, -159.6898) -> (-268.1697, -159.6898)
  line L25 (-268.1697, -159.6898) -> (-268.1697, -154.6898)
  line L26 (-268.1697, -154.6898) -> (-281.8061, -154.6898)
  line L27 (-281.8061, -154.6898) -> (-281.8061, -159.6898)
  line L28 (-281.8061, -159.6898) -> (-295.4424, -159.6898)
  line L29 (-295.4424, -159.6898) -> (-295.4424, -154.6898)
  line L30 (-295.4424, -154.6898) -> (-309.0788, -154.6898)
  line L31 (-309.0788, -154.6898) -> (-309.0788, -159.6898)
  line L32 (-309.0788, -159.6898) -> (-322.7151, -159.6898)
  line L33 (-322.7151, -159.6898) -> (-322.7151, -176.6898)
  line L34 (-322.7151, -176.6898) -> (-317.7151, -176.6898)
  line L35 (-317.7151, -176.6898) -> (-317.7151, -198.6898)
  line L36 (-317.7151, -198.6898) -> (-322.7151, -198.6898)
  line L37 (-322.7151, -198.6898) -> (-322.7151, -220.6898)
  line L38 (-322.7151, -220.6898) -> (-317.7151, -220.6898)
  line L39 (-317.7151, -220.6898) -> (-317.7151, -242.6898)
sketch "Sketch12" plane through (150, 0, 0) normal (1, 0, 0) x (0, 1, 0)
sketch "Sketch13" plane through (0, 0, 0) normal (1, 0, 0) x (0, 1, 0)
  circle A0 centre (-285.2151, -228.0231) radius 7.5
  circle A1 centre (-260.2151, -228.0231) radius 7.5
  circle A2 centre (-235.2151, -228.0231) radius 7.5
  circle A3 centre (-210.2151, -228.0231) radius 7.5
  line L0 (-317.7151, -242.6898) -> (-322.7151, -242.6898)
  line L1 (-322.7151, -242.6898) -> (-322.7151, -264.6898)
  line L2 (-322.7151, -264.6898) -> (-172.7151, -264.6898)
  line L3 (-172.7151, -264.6898) -> (-172.7151, -242.6898)
  line L4 (-172.7151, -242.6898) -> (-177.7151, -242.6898)
  line L5 (-177.7151, -242.6898) -> (-177.7151, -220.6898)
  line L6 (-177.7151, -220.6898) -> (-172.7151, -220.6898)
  line L7 (-172.7151, -220.6898) -> (-172.7151, -198.6898)
  line L8 (-172.7151, -198.6898) -> (-177.7151, -198.6898)
  line L9 (-177.7151, -198.6898) -> (-177.7151, -176.6898)
  line L10 (-177.7151, -176.6898) -> (-172.7151, -176.6898)
  line L11 (-172.7151, -176.6898) -> (-172.7151, -159.6898)
  line L12 (-172.7151, -159.6898) -> (-186.3515, -159.6898)
  line L13 (-186.3515, -159.6898) -> (-186.3515, -154.6898)
  line L14 (-186.3515, -154.6898) -> (-199.9879, -154.6898)
  line L15 (-199.9879, -154.6898) -> (-199.9879, -159.6898)
  line L16 (-199.9879, -159.6898) -> (-213.6242, -159.6898)
  line L17 (-213.6242, -159.6898) -> (-213.6242, -154.6898)
  line L18 (-213.6242, -154.6898) -> (-227.2606, -154.6898)
  line L19 (-227.2606, -154.6898) -> (-227.2606, -159.6898)
  line L20 (-227.2606, -159.6898) -> (-240.897, -159.6898)
  line L21 (-240.897, -159.6898) -> (-240.897, -154.6898)
  line L22 (-240.897, -154.6898) -> (-254.5333, -154.6898)
  line L23 (-254.5333, -154.6898) -> (-254.5333, -159.6898)
  line L24 (-254.5333, -159.6898) -> (-268.1697, -159.6898)
  line L25 (-268.1697, -159.6898) -> (-268.1697, -154.6898)
  line L26 (-268.1697, -154.6898) -> (-281.8061, -154.6898)
  line L27 (-281.8061, -154.6898) -> (-281.8061, -159.6898)
  line L28 (-281.8061, -159.6898) -> (-295.4424, -159.6898)
  line L29 (-295.4424, -159.6898) -> (-295.4424, -154.6898)
  line L30 (-295.4424, -154.6898) -> (-309.0788, -154.6898)
  line L31 (-309.0788, -154.6898) -> (-309.0788, -159.6898)
  line L32 (-309.0788, -159.6898) -> (-322.7151, -159.6898)
  line L33 (-322.7151, -159.6898) -> (-322.7151, -176.6898)
  line L34 (-322.7151, -176.6898) -> (-317.7151, -176.6898)
  line L35 (-317.7151, -176.6898) -> (-317.7151, -198.6898)
  line L36 (-317.7151, -198.6898) -> (-322.7151, -198.6898)
  line L37 (-322.7151, -198.6898) -> (-322.7151, -220.6898)
  line L38 (-322.7151, -220.6898) -> (-317.7151, -220.6898)
  line L39 (-317.7151, -220.6898) -> (-317.7151, -242.6898)
  line L40 (-150.2242, -159.4799) -> (-163.1131, -159.4799)
  line L41 (-163.1131, -159.4799) -> (-163.1131, -176.4799)
  line L42 (-163.1131, -176.4799) -> (-168.1131, -176.4799)
  line L43 (-168.1131, -176.4799) -> (-168.1131, -198.4799)
  line L44 (-168.1131, -198.4799) -> (-163.1131, -198.4799)
  line L45 (-163.1131, -198.4799) -> (-163.1131, -220.4799)
  line L46 (-163.1131, -220.4799) -> (-168.1131, -220.4799)
  line L47 (-168.1131, -220.4799) -> (-168.1131, -242.4799)
  line L48 (-168.1131, -242.4799) -> (-163.1131, -242.4799)
  line L49 (-163.1131, -242.4799) -> (-163.1131, -264.4799)
  line L50 (-163.1131, -264.4799) -> (-12.1131, -264.4799)
  line L51 (-12.1131, -264.4799) -> (-12.1131, -242.4799)
  line L52 (-12.1131, -242.4799) -> (-7.1131, -242.4799)
  line L53 (-7.1131, -242.4799) -> (-7.1131, -220.4799)
  line L54 (-7.1131, -220.4799) -> (-12.1131, -220.4799)
  line L55 (-12.1131, -220.4799) -> (-12.1131, -198.4799)
  line L56 (-12.1131, -198.4799) -> (-7.1131, -198.4799)
  line L57 (-7.1131, -198.4799) -> (-7.1131, -176.4799)
  line L58 (-7.1131, -176.4799) -> (-12.1131, -176.4799)
  line L59 (-12.1131, -176.4799) -> (-12.1131, -159.4799)
  line L60 (-12.1131, -159.4799) -> (-25.002, -159.4799)
  line L61 (-25.002, -159.4799) -> (-25.002, -154.4799)
  line L62 (-25.002, -154.4799) -> (-42.8909, -154.4799)
  line L63 (-42.8909, -154.4799) -> (-42.8909, -159.4799)
  line L64 (-42.8909, -159.4799) -> (-60.7798, -159.4799)
  line L65 (-60.7798, -159.4799) -> (-60.7798, -154.4799)
  line L66 (-60.7798, -154.4799) -> (-78.6687, -154.4799)
  line L67 (-78.6687, -154.4799) -> (-78.6687, -159.4799)
  line L68 (-78.6687, -159.4799) -> (-96.5576, -159.4799)
  line L69 (-96.5576, -159.4799) -> (-96.5576, -154.4799)
  line L70 (-96.5576, -154.4799) -> (-114.4464, -154.4799)
  line L71 (-114.4464, -154.4799) -> (-114.4464, -159.4799)
  line L72 (-114.4464, -159.4799) -> (-132.3353, -159.4799)
  line L73 (-132.3353, -159.4799) -> (-132.3353, -154.4799)
  line L74 (-132.3353, -154.4799) -> (-150.2242, -154.4799)
  line L75 (-150.2242, -154.4799) -> (-150.2242, -159.4799)
  line L76 (-54.7798, -175.9799) -> (-54.7798, -181.9799)
  line L77 (-54.7798, -181.9799) -> (-60.7798, -181.9799)
  line L78 (-60.7798, -181.9799) -> (-60.7798, -175.9799)
  line L79 (-60.7798, -175.9799) -> (-54.7798, -175.9799)
  line L80 (-62.4464, -175.9799) -> (-62.4464, -181.9799)
  line L81 (-62.4464, -181.9799) -> (-68.4464, -181.9799)
  line L82 (-68.4464, -181.9799) -> (-68.4464, -175.9799)
  line L83 (-68.4464, -175.9799) -> (-62.4464, -175.9799)
  line L84 (-70.1131, -175.9799) -> (-70.1131, -181.9799)
  line L85 (-70.1131, -181.9799) -> (-76.1131, -181.9799)
  line L86 (-76.1131, -181.9799) -> (-76.1131, -175.9799)
  line L87 (-76.1131, -175.9799) -> (-70.1131, -175.9799)
  line L88 (-77.7798, -175.9799) -> (-77.7798, -181.9799)
  line L89 (-77.7798, -181.9799) -> (-83.7798, -181.9799)
  line L90 (-83.7798, -181.9799) -> (-83.7798, -175.9799)
  line L91 (-83.7798, -175.9799) -> (-77.7798, -175.9799)
  line L92 (-85.4464, -175.9799) -> (-85.4464, -181.9799)
  line L93 (-85.4464, -181.9799) -> (-91.4464, -181.9799)
  line L94 (-91.4464, -181.9799) -> (-91.4464, -175.9799)
  line L95 (-91.4464, -175.9799) -> (-85.4464, -175.9799)
  line L96 (-93.1131, -175.9799) -> (-93.1131, -181.9799)
  line L97 (-93.1131, -181.9799) -> (-99.1131, -181.9799)
  line L98 (-99.1131, -181.9799) -> (-99.1131, -175.9799)
  line L99 (-99.1131, -175.9799) -> (-93.1131, -175.9799)
  line L100 (-100.7798, -175.9799) -> (-100.7798, -181.9799)
  line L101 (-100.7798, -181.9799) -> (-106.7798, -181.9799)
  line L102 (-106.7798, -181.9799) -> (-106.7798, -175.9799)
  line L103 (-106.7798, -175.9799) -> (-100.7798, -175.9799)
  line L104 (-108.4464, -175.9799) -> (-108.4464, -181.9799)
  line L105 (-108.4464, -181.9799) -> (-114.4464, -181.9799)
  line L106 (-114.4464, -181.9799) -> (-114.4464, -175.9799)
  line L107 (-114.4464, -175.9799) -> (-108.4464, -175.9799)
  line L108 (-54.7798, -183.837) -> (-54.7798, -189.837)
  line L109 (-54.7798, -189.837) -> (-60.7798, -189.837)
  line L110 (-60.7798, -189.837) -> (-60.7798, -183.837)
  line L111 (-60.7798, -183.837) -> (-54.7798, -183.837)
  line L112 (-62.4464, -183.837) -> (-62.4464, -189.837)
  line L113 (-62.4464, -189.837) -> (-68.4464, -189.837)
  line L114 (-68.4464, -189.837) -> (-68.4464, -183.837)
  line L115 (-68.4464, -183.837) -> (-62.4464, -183.837)
  line L116 (-70.1131, -183.837) -> (-70.1131, -189.837)
  line L117 (-70.1131, -189.837) -> (-76.1131, -189.837)
  line L118 (-76.1131, -189.837) -> (-76.1131, -183.837)
  line L119 (-76.1131, -183.837) -> (-70.1131, -183.837)
  line L120 (-77.7798, -183.837) -> (-77.7798, -189.837)
  line L121 (-77.7798, -189.837) -> (-83.7798, -189.837)
  line L122 (-83.7798, -189.837) -> (-83.7798, -183.837)
  line L123 (-83.7798, -183.837) -> (-77.7798, -183.837)
  line L124 (-85.4464, -183.837) -> (-85.4464, -189.837)
  line L125 (-85.4464, -189.837) -> (-91.4464, -189.837)
  line L126 (-91.4464, -189.837) -> (-91.4464, -183.837)
  line L127 (-91.4464, -183.837) -> (-85.4464, -183.837)
  line L128 (-93.1131, -183.837) -> (-93.1131, -189.837)
  line L129 (-93.1131, -189.837) -> (-99.1131, -189.837)
  line L130 (-99.1131, -189.837) -> (-99.1131, -183.837)
  line L131 (-99.1131, -183.837) -> (-93.1131, -183.837)
  line L132 (-100.7798, -183.837) -> (-100.7798, -189.837)
  line L133 (-100.7798, -189.837) -> (-106.7798, -189.837)
  line L134 (-106.7798, -189.837) -> (-106.7798, -183.837)
  line L135 (-106.7798, -183.837) -> (-100.7798, -183.837)
  line L136 (-108.4464, -183.837) -> (-108.4464, -189.837)
  line L137 (-108.4464, -189.837) -> (-114.4464, -189.837)
  line L138 (-114.4464, -189.837) -> (-114.4464, -183.837)
  line L139 (-114.4464, -183.837) -> (-108.4464, -183.837)
  line L140 (-54.7798, -191.6942) -> (-54.7798, -197.6942)
  line L141 (-54.7798, -197.6942) -> (-60.7798, -197.6942)
  line L142 (-60.7798, -197.6942) -> (-60.7798, -191.6942)
  line L143 (-60.7798, -191.6942) -> (-54.7798, -191.6942)
  line L144 (-62.4464, -191.6942) -> (-62.4464, -197.6942)
  line L145 (-62.4464, -197.6942) -> (-68.4464, -197.6942)
  line L146 (-68.4464, -197.6942) -> (-68.4464, -191.6942)
  line L147 (-68.4464, -191.6942) -> (-62.4464, -191.6942)
  line L148 (-70.1131, -191.6942) -> (-70.1131, -197.6942)
  line L149 (-70.1131, -197.6942) -> (-76.1131, -197.6942)
  line L150 (-76.1131, -197.6942) -> (-76.1131, -191.6942)
  line L151 (-76.1131, -191.6942) -> (-70.1131, -191.6942)
  line L152 (-77.7798, -191.6942) -> (-77.7798, -197.6942)
  line L153 (-77.7798, -197.6942) -> (-83.7798, -197.6942)
  line L154 (-83.7798, -197.6942) -> (-83.7798, -191.6942)
  line L155 (-83.7798, -191.6942) -> (-77.7798, -191.6942)
  line L156 (-85.4464, -191.6942) -> (-85.4464, -197.6942)
  line L157 (-85.4464, -197.6942) -> (-91.4464, -197.6942)
  line L158 (-91.4464, -197.6942) -> (-91.4464, -191.6942)
  line L159 (-91.4464, -191.6942) -> (-85.4464, -191.6942)
  line L160 (-93.1131, -191.6942) -> (-93.1131, -197.6942)
  line L161 (-93.1131, -197.6942) -> (-99.1131, -197.6942)
  line L162 (-99.1131, -197.6942) -> (-99.1131, -191.6942)
  line L163 (-99.1131, -191.6942) -> (-93.1131, -191.6942)
  line L164 (-100.7798, -191.6942) -> (-100.7798, -197.6942)
  line L165 (-100.7798, -197.6942) -> (-106.7798, -197.6942)
  line L166 (-106.7798, -197.6942) -> (-106.7798, -191.6942)
  line L167 (-106.7798, -191.6942) -> (-100.7798, -191.6942)
  line L168 (-108.4464, -191.6942) -> (-108.4464, -197.6942)
  line L169 (-108.4464, -197.6942) -> (-114.4464, -197.6942)
  line L170 (-114.4464, -197.6942) -> (-114.4464, -191.6942)
  line L171 (-114.4464, -191.6942) -> (-108.4464, -191.6942)
  line L172 (-54.7798, -199.5513) -> (-54.7798, -205.5513)
  line L173 (-54.7798, -205.5513) -> (-60.7798, -205.5513)
  line L174 (-60.7798, -205.5513) -> (-60.7798, -199.5513)
  line L175 (-60.7798, -199.5513) -> (-54.7798, -199.5513)
  line L176 (-62.4464, -199.5513) -> (-62.4464, -205.5513)
  line L177 (-62.4464, -205.5513) -> (-68.4464, -205.5513)
  line L178 (-68.4464, -205.5513) -> (-68.4464, -199.5513)
  line L179 (-68.4464, -199.5513) -> (-62.4464, -199.5513)
  line L180 (-70.1131, -199.5513) -> (-70.1131, -205.5513)
  line L181 (-70.1131, -205.5513) -> (-76.1131, -205.5513)
  line L182 (-76.1131, -205.5513) -> (-76.1131, -199.5513)
  line L183 (-76.1131, -199.5513) -> (-70.1131, -199.5513)
  line L184 (-77.7798, -199.5513) -> (-77.7798, -205.5513)
  line L185 (-77.7798, -205.5513) -> (-83.7798, -205.5513)
  line L186 (-83.7798, -205.5513) -> (-83.7798, -199.5513)
  line L187 (-83.7798, -199.5513) -> (-77.7798, -199.5513)
  line L188 (-85.4464, -199.5513) -> (-85.4464, -205.5513)
  line L189 (-85.4464, -205.5513) -> (-91.4464, -205.5513)
  line L190 (-91.4464, -205.5513) -> (-91.4464, -199.5513)
  line L191 (-91.4464, -199.5513) -> (-85.4464, -199.5513)
  line L192 (-93.1131, -199.5513) -> (-93.1131, -205.5513)
  line L193 (-93.1131, -205.5513) -> (-99.1131, -205.5513)
  line L194 (-99.1131, -205.5513) -> (-99.1131, -199.5513)
  line L195 (-99.1131, -199.5513) -> (-93.1131, -199.5513)
  line L196 (-100.7798, -199.5513) -> (-100.7798, -205.5513)
  line L197 (-100.7798, -205.5513) -> (-106.7798, -205.5513)
  line L198 (-106.7798, -205.5513) -> (-106.7798, -199.5513)
  line L199 (-106.7798, -199.5513) -> (-100.7798, -199.5513)
  line L200 (-108.4464, -199.5513) -> (-108.4464, -205.5513)
  line L201 (-108.4464, -205.5513) -> (-114.4464, -205.5513)
  line L202 (-114.4464, -205.5513) -> (-114.4464, -199.5513)
  line L203 (-114.4464, -199.5513) -> (-108.4464, -199.5513)
  line L204 (-54.7798, -207.4085) -> (-54.7798, -213.4085)
  line L205 (-54.7798, -213.4085) -> (-60.7798, -213.4085)
  line L206 (-60.7798, -213.4085) -> (-60.7798, -207.4085)
  line L207 (-60.7798, -207.4085) -> (-54.7798, -207.4085)
  line L208 (-62.4464, -207.4085) -> (-62.4464, -213.4085)
  line L209 (-62.4464, -213.4085) -> (-68.4464, -213.4085)
  line L210 (-68.4464, -213.4085) -> (-68.4464, -207.4085)
  line L211 (-68.4464, -207.4085) -> (-62.4464, -207.4085)
  line L212 (-70.1131, -207.4085) -> (-70.1131, -213.4085)
  line L213 (-70.1131, -213.4085) -> (-76.1131, -213.4085)
  line L214 (-76.1131, -213.4085) -> (-76.1131, -207.4085)
  line L215 (-76.1131, -207.4085) -> (-70.1131, -207.4085)
  line L216 (-77.7798, -207.4085) -> (-77.7798, -213.4085)
  line L217 (-77.7798, -213.4085) -> (-83.7798, -213.4085)
  line L218 (-83.7798, -213.4085) -> (-83.7798, -207.4085)
  line L219 (-83.7798, -207.4085) -> (-77.7798, -207.4085)
  line L220 (-85.4464, -207.4085) -> (-85.4464, -213.4085)
  line L221 (-85.4464, -213.4085) -> (-91.4464, -213.4085)
  line L222 (-91.4464, -213.4085) -> (-91.4464, -207.4085)
  line L223 (-91.4464, -207.4085) -> (-85.4464, -207.4085)
  line L224 (-93.1131, -207.4085) -> (-93.1131, -213.4085)
  line L225 (-93.1131, -213.4085) -> (-99.1131, -213.4085)
  line L226 (-99.1131, -213.4085) -> (-99.1131, -207.4085)
  line L227 (-99.1131, -207.4085) -> (-93.1131, -207.4085)
  line L228 (-100.7798, -207.4085) -> (-100.7798, -213.4085)
  line L229 (-100.7798, -213.4085) -> (-106.7798, -213.4085)
  line L230 (-106.7798, -213.4085) -> (-106.7798, -207.4085)
  line L231 (-106.7798, -207.4085) -> (-100.7798, -207.4085)
  line L232 (-108.4464, -207.4085) -> (-108.4464, -213.4085)
  line L233 (-108.4464, -213.4085) -> (-114.4464, -213.4085)
  line L234 (-114.4464, -213.4085) -> (-114.4464, -207.4085)
  line L235 (-114.4464, -207.4085) -> (-108.4464, -207.4085)
  line L236 (-54.7798, -215.2656) -> (-54.7798, -221.2656)
  line L237 (-54.7798, -221.2656) -> (-60.7798, -221.2656)
  line L238 (-60.7798, -221.2656) -> (-60.7798, -215.2656)
  line L239 (-60.7798, -215.2656) -> (-54.7798, -215.2656)
  line L240 (-62.4464, -215.2656) -> (-62.4464, -221.2656)
  line L241 (-62.4464, -221.2656) -> (-68.4464, -221.2656)
  line L242 (-68.4464, -221.2656) -> (-68.4464, -215.2656)
  line L243 (-68.4464, -215.2656) -> (-62.4464, -215.2656)
  line L244 (-70.1131, -215.2656) -> (-70.1131, -221.2656)
  line L245 (-70.1131, -221.2656) -> (-76.1131, -221.2656)
  line L246 (-76.1131, -221.2656) -> (-76.1131, -215.2656)
  line L247 (-76.1131, -215.2656) -> (-70.1131, -215.2656)
  line L248 (-77.7798, -215.2656) -> (-77.7798, -221.2656)
  line L249 (-77.7798, -221.2656) -> (-83.7798, -221.2656)
  line L250 (-83.7798, -221.2656) -> (-83.7798, -215.2656)
  line L251 (-83.7798, -215.2656) -> (-77.7798, -215.2656)
  line L252 (-85.4464, -215.2656) -> (-85.4464, -221.2656)
  line L253 (-85.4464, -221.2656) -> (-91.4464, -221.2656)
  line L254 (-91.4464, -221.2656) -> (-91.4464, -215.2656)
  line L255 (-91.4464, -215.2656) -> (-85.4464, -215.2656)
  line L256 (-93.1131, -215.2656) -> (-93.1131, -221.2656)
  line L257 (-93.1131, -221.2656) -> (-99.1131, -221.2656)
  line L258 (-99.1131, -221.2656) -> (-99.1131, -215.2656)
  line L259 (-99.1131, -215.2656) -> (-93.1131, -215.2656)
  line L260 (-100.7798, -215.2656) -> (-100.7798, -221.2656)
  line L261 (-100.7798, -221.2656) -> (-106.7798, -221.2656)
  line L262 (-106.7798, -221.2656) -> (-106.7798, -215.2656)
  line L263 (-106.7798, -215.2656) -> (-100.7798, -215.2656)
  line L264 (-108.4464, -215.2656) -> (-108.4464, -221.2656)
  line L265 (-108.4464, -221.2656) -> (-114.4464, -221.2656)
  line L266 (-114.4464, -221.2656) -> (-114.4464, -215.2656)
  line L267 (-114.4464, -215.2656) -> (-108.4464, -215.2656)
  line L268 (-54.7798, -223.1228) -> (-54.7798, -229.1228)
  line L269 (-54.7798, -229.1228) -> (-60.7798, -229.1228)
  line L270 (-60.7798, -229.1228) -> (-60.7798, -223.1228)
  line L271 (-60.7798, -223.1228) -> (-54.7798, -223.1228)
  line L272 (-62.4464, -223.1228) -> (-62.4464, -229.1228)
  line L273 (-62.4464, -229.1228) -> (-68.4464, -229.1228)
  line L274 (-68.4464, -229.1228) -> (-68.4464, -223.1228)
  line L275 (-68.4464, -223.1228) -> (-62.4464, -223.1228)
  line L276 (-70.1131, -223.1228) -> (-70.1131, -229.1228)
  line L277 (-70.1131, -229.1228) -> (-76.1131, -229.1228)
  line L278 (-76.1131, -229.1228) -> (-76.1131, -223.1228)
  line L279 (-76.1131, -223.1228) -> (-70.1131, -223.1228)
  line L280 (-77.7798, -223.1228) -> (-77.7798, -229.1228)
  line L281 (-77.7798, -229.1228) -> (-83.7798, -229.1228)
  line L282 (-83.7798, -229.1228) -> (-83.7798, -223.1228)
  line L283 (-83.7798, -223.1228) -> (-77.7798, -223.1228)
  line L284 (-85.4464, -223.1228) -> (-85.4464, -229.1228)
  line L285 (-85.4464, -229.1228) -> (-91.4464, -229.1228)
  line L286 (-91.4464, -229.1228) -> (-91.4464, -223.1228)
  line L287 (-91.4464, -223.1228) -> (-85.4464, -223.1228)
  line L288 (-93.1131, -223.1228) -> (-93.1131, -229.1228)
  line L289 (-93.1131, -229.1228) -> (-99.1131, -229.1228)
  line L290 (-99.1131, -229.1228) -> (-99.1131, -223.1228)
  line L291 (-99.1131, -223.1228) -> (-93.1131, -223.1228)
  line L292 (-100.7798, -223.1228) -> (-100.7798, -229.1228)
  line L293 (-100.7798, -229.1228) -> (-106.7798, -229.1228)
  line L294 (-106.7798, -229.1228) -> (-106.7798, -223.1228)
  line L295 (-106.7798, -223.1228) -> (-100.7798, -223.1228)
  line L296 (-108.4464, -223.1228) -> (-108.4464, -229.1228)
  line L297 (-108.4464, -229.1228) -> (-114.4464, -229.1228)
  line L298 (-114.4464, -229.1228) -> (-114.4464, -223.1228)
  line L299 (-114.4464, -223.1228) -> (-108.4464, -223.1228)
  line L300 (-54.7798, -230.9799) -> (-54.7798, -236.9799)
  line L301 (-54.7798, -236.9799) -> (-60.7798, -236.9799)
  line L302 (-60.7798, -236.9799) -> (-60.7798, -230.9799)
  line L303 (-60.7798, -230.9799) -> (-54.7798, -230.9799)
  line L304 (-62.4464, -230.9799) -> (-62.4464, -236.9799)
  line L305 (-62.4464, -236.9799) -> (-68.4464, -236.9799)
  line L306 (-68.4464, -236.9799) -> (-68.4464, -230.9799)
  line L307 (-68.4464, -230.9799) -> (-62.4464, -230.9799)
  line L308 (-70.1131, -230.9799) -> (-70.1131, -236.9799)
  line L309 (-70.1131, -236.9799) -> (-76.1131, -236.9799)
  line L310 (-76.1131, -236.9799) -> (-76.1131, -230.9799)
  line L311 (-76.1131, -230.9799) -> (-70.1131, -230.9799)
  line L312 (-77.7798, -230.9799) -> (-77.7798, -236.9799)
  line L313 (-77.7798, -236.9799) -> (-83.7798, -236.9799)
  line L314 (-83.7798, -236.9799) -> (-83.7798, -230.9799)
  line L315 (-83.7798, -230.9799) -> (-77.7798, -230.9799)
  line L316 (-85.4464, -230.9799) -> (-85.4464, -236.9799)
  line L317 (-85.4464, -236.9799) -> (-91.4464, -236.9799)
  line L318 (-91.4464, -236.9799) -> (-91.4464, -230.9799)
  line L319 (-91.4464, -230.9799) -> (-85.4464, -230.9799)
  line L320 (-93.1131, -230.9799) -> (-93.1131, -236.9799)
  line L321 (-93.1131, -236.9799) -> (-99.1131, -236.9799)
  line L322 (-99.1131, -236.9799) -> (-99.1131, -230.9799)
  line L323 (-99.1131, -230.9799) -> (-93.1131, -230.9799)
  line L324 (-100.7798, -230.9799) -> (-100.7798, -236.9799)
  line L325 (-100.7798, -236.9799) -> (-106.7798, -236.9799)
  line L326 (-106.7798, -236.9799) -> (-106.7798, -230.9799)
  line L327 (-106.7798, -230.9799) -> (-100.7798, -230.9799)